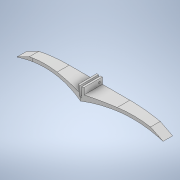
# Autodesk Inventor part: пиналка_верх
Saved by Autodesk Inventor 2020 (Build 240168000, 168)
## iProperties
Created: 2025-01-29
Part Number: пиналка_верх
Material: Типовые
Document SubType Name: Modeling
Designer: frozj
Density: 1 g/cm^3
Appearance: По умолчанию
Author: frozj
Autodesk Inventor part; units mm, degrees
ref_plane "YZ Plane" through (0, 0, 0) normal (1, 0, 0) x (0, 1, 0)
ref_plane "XZ Plane" through (0, 0, 0) normal (0, 1, 0) x (-1, 0, 0)
ref_plane "XY Plane" through (0, 0, 0) normal (0, 0, 1) x (1, 0, 0)
sketch "Эскиз1" plane through (0, 0, 0) normal (0, 0, 1) x (1, 0, 0)
  line L0 (115, 5) -> (-115, 5)
  line L1 (-115, 5) -> (-115, -5)
  line L2 (-115, -5) -> (115, -5)
  line L3 (115, -5) -> (115, 5)
  line L4 (115, 5) -> (-115, -5) construction
  line L5 (-115, 5) -> (115, -5) construction
  arc A0 (0, 0) -> (-115, -5) centre (-47.7882, -225.8713) ccw
  arc A1 (115, -5) -> (0, 0) centre (47.7882, -225.8713) ccw
  line L6 (115, 10) -> (-115, 10)
  line L7 (-115, 10) -> (-115, 0)
  line L8 (-115, 0) -> (115, 0)
  line L9 (115, 0) -> (115, 10)
  line L10 (115, 10) -> (-115, 0) construction
  line L11 (-115, 10) -> (115, 0) construction
  arc A2 (0, 5) -> (-115, 0) centre (-47.7882, -220.8713) ccw
  arc A3 (115, 0) -> (0, 5) centre (47.7882, -220.8713) ccw
  line L12 (-115, -5) -> (-95.5764, 5)
  line L13 (115, -5) -> (95.5764, 5)
  line L14 (1.5, 15) -> (-1.5, 15)
  line L15 (-1.5, 15) -> (-1.5, -5)
  line L16 (-1.5, -5) -> (1.5, -5)
  line L17 (1.5, -5) -> (1.5, 15)
  line L18 (1.5, 15) -> (-1.5, -5) construction
  line L19 (-1.5, 15) -> (1.5, -5) construction
  line L20 (-1.5, 5) -> (1.5, 5)
  line L21 (1.5, 5) -> (1.5, 20)
  line L22 (1.5, 20) -> (-1.5, 20)
  line L23 (-1.5, 20) -> (-1.5, 5)
  circle A4 centre (0, 15) radius 1.5
  line L24 (1.5, 20) -> (4.5, 20)
  line L25 (4.5, 20) -> (4.5, 5)
  line L26 (4.5, 5) -> (1.5, 5)
  line L27 (1.5, 5) -> (1.5, 20)
  line L28 (-1.5, 20) -> (-4.5, 20)
  line L29 (-4.5, 20) -> (-4.5, 5)
  line L30 (-4.5, 5) -> (-1.5, 5)
  line L31 (-1.5, 5) -> (-1.5, 20)
  line L32 (-47.7882, 10) -> (-4.5, 10)
  line L33 (4.5, 10) -> (47.7882, 10)
  line L34 (4.5, 13.5) -> (-4.5, 13.5)
  line L35 (-4.5, 13.5) -> (-4.5, 16.5)
  line L36 (-4.5, 16.5) -> (4.5, 16.5)
  line L37 (4.5, 16.5) -> (4.5, 13.5)
  line L38 (4.5, 13.5) -> (-4.5, 16.5) construction
  line L39 (-4.5, 13.5) -> (4.5, 16.5) construction
  line L40 (4.5, 12.5) -> (-4.5, 12.5)
  line L41 (-4.5, 12.5) -> (-4.5, 17.5)
  line L42 (-4.5, 17.5) -> (4.5, 17.5)
  line L43 (4.5, 17.5) -> (4.5, 12.5)
  line L44 (4.5, 12.5) -> (-4.5, 17.5) construction
  line L45 (-4.5, 12.5) -> (4.5, 17.5) construction
  point P0 (1.5, 5.3122)
  point P1 (4.5, 5.9054)
  point P2 (-4.5, 5.9054)
  point P3 (-1.5, 5.3122)
  dimension "d6" = 3
  dimension "d0" = 230
  dimension "d1" = 10
  dimension "d4" = 3
  dimension "d5" = 15
  dimension "d7" = 3
  dimension "d8" = 3
  dimension "d9" = 5
  constraints: 92 end point, 16 parallel, 14 midpoint, 13 point on line, 12 point on circle, 8 horizontal, 8 perpendicular, 4 centre point, 4 tangent, 1 horizontal alignment, 2 other
  measures "d0" distance of L2.end L1.end
  measures "d1" distance of L1.end L0.end
  measures "d4" distance of L16.end L15.end
  measures "d5" distance of L21.end L20.end
  measures "d7" distance of L25.end L26.end
  measures "d8" distance of L30.end L29.end
  measures "d9" distance of L40.end L41.end
extrude "Выдавливание1" add sketch "Эскиз1" along normal blind 30 contours L13 L8 A1 L0 | L0 L25 A3 | A1 L17 L0 | A3 L25 L6 | L13 A1 L8 | L0 L17 A3 L25 | A1 A0 L15 L0 L17 | L25 A3 L17 L6 | L6 L17 L40 L25 | L40 L17 L34 L25 | A0 L0 L15 | L15 A2 L29 L6 | L6 L29 L40 L15 | L34 L17 L21 L36 L25 | L12 L8 A0 | L0 L29 A2 L15 | L0 A2 L29 | A0 L8 L12 L0 | L29 A2 L6 | L40 L29 L34 L15 | L36 L21 L42 L25 | L34 L29 L36 L23 L15 | L42 L21 L24 L25 | L29 L42 L23 L36 | L42 L29 L28 L23
sketch "Эскиз2" plane through (0, 0, 0) normal (0, 1, 0) x (-1, 0, 0)
  line L0 (115, 0) -> (0, 0) projected
  line L1 (0, 0) -> (0, 30) projected
  line L2 (115, 30) -> (0, 30) projected
  line L3 (115, 0) -> (115, 30) projected
  line L4 (0, 0) -> (-115, 0) projected
  line L5 (-115, 0) -> (-115, 30) projected
  line L6 (0, 30) -> (-115, 30) projected
  line L7 (0, 0) -> (0, 30) projected
  line L8 (95.5764, 0) -> (115, 0) projected
  line L9 (-115, 0) -> (-115, 30) projected
  line L10 (115, 0) -> (-115, 0)
  line L11 (-115, 0) -> (-115, 15)
  line L12 (-115, 15) -> (115, 15)
  line L13 (115, 15) -> (115, 0)
  line L14 (0, 0) -> (0, 30) projected
  arc A0 (0, 30) -> (115, 15) centre (102.5177, 367.6359) ccw
  arc A1 (-115, 15) -> (0, 30) centre (-111.4518, 436.1301) ccw
  point P0 (90.0355, 15)
  point P1 (-107.9035, 15)
  constraints: 8 end point, 4 point on circle, 2 centre point, 2 parallel, 1 horizontal, 1 midpoint, 1 perpendicular
extrude "Выдавливание2" cut sketch "Эскиз2" along normal mid plane 40 contours L12 A0 L2 L3 | A1 L12 L5 L6
sketch "Эскиз7" plane through (-4.5, 10, 0) normal (-1, 0, 0) x (0, 0, 1)
  line L0 (0, 10) -> (28.6663, 10) projected
  line L1 (0, 10) -> (5, 10)
  line L2 (5, 10) -> (5, 5)
  line L3 (5, 5) -> (0, 5)
  line L4 (0, 5) -> (0, 10)
  circle A0 centre (5, 5) radius 1.5
  point P0 (0, -10)
  dimension "d68" = 5
  dimension "d69" = 5
  dimension "d70" = 3
  constraints: 8 end point, 2 parallel, 1 centre point, 1 coincident, 1 horizontal, 1 perpendicular
  measures "d68" distance of L2.end L3.end
  measures "d69" distance of L1.end L2.end
  measures "d70" diameter of A0
extrude "Выдавливание7" cut sketch "Эскиз7" against normal blind 40 contours A0 L3 L2 | L2 L3 A0
